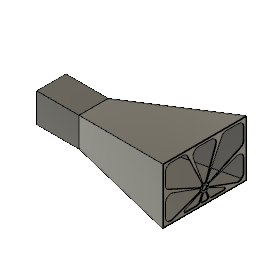
ion thruster-4 v1 (Autodesk Fusion 360 design; units mm, degrees)
Autodesk Fusion 360 part; units mm, degrees
sketch "Skizze7" plane through (0, 0, 0) normal (1, 0, 0) x (0, 1, 0)
  line L0 (-53, 53) -> (53, 53)
  line L1 (53, 53) -> (53, -53)
  line L2 (53, -53) -> (-53, -53)
  line L3 (-53, -53) -> (-53, 53)
  line L4 (-53, 53) -> (53, -53) construction
  line L5 (53, 53) -> (-53, -53) construction
  dimension "d31" = 106
  dimension "d32" = 106
  constraint horizontal L0
  constraint perpendicular L0 L1
  constraint parallel L0 L2
  constraint parallel L1 L3
  constraint coincident L4 origin
  constraint coincident L5 origin
  measures "d31" distance of L1.end L2.end
  measures "d32" distance of L0.end L1.end
extrude "Extrusion4" add sketch "Skizze7" against normal blind 153 makes body 1
sketch "Skizze8" plane through (0, 0, 0) normal (1, 0, 0) x (0, 1, 0)
  line L0 (50, -50) -> (-50, -50)
  line L1 (-50, -50) -> (-50, 50)
  line L2 (-50, 50) -> (50, 50)
  line L3 (50, 50) -> (50, -50)
  line L4 (50, -50) -> (-50, 50) construction
  line L5 (-50, -50) -> (50, 50) construction
  dimension "d35" = 100
  dimension "d36" = 100
  constraint horizontal L0
  constraint perpendicular L0 L1
  constraint parallel L0 L2
  constraint parallel L1 L3
  constraint coincident L4 origin
  constraint coincident L5 origin
  measures "d35" distance of L1.end L2.end
  measures "d36" distance of L0.end L1.end
extrude "Extrusion5" cut sketch "Skizze8" against normal blind 150 bodies 1
sketch "Skizze9" plane through (-153, 0, 0) normal (-1, 0, 0) x (0, -1, 0)
  line L0 (-53, -53) -> (53, -53)
  line L1 (53, -53) -> (53, 53)
  line L2 (53, 53) -> (-53, 53)
  line L3 (-53, 53) -> (-53, -53)
  line L4 (53, 53) -> (-53, 53)
  line L5 (-53, 53) -> (-53, -53)
  line L6 (-53, -53) -> (53, -53)
  line L7 (53, -53) -> (53, 53)
  circle A0 centre (0, 0) radius 9
  line L8 (-6.1659, -16.9405) -> (-14.5398, -39.9479)
  line L9 (-16.2488, -5.9141) -> (-39.9479, -14.5398)
  line L10 (-16.9405, 6.1659) -> (-39.9479, 14.5398)
  line L11 (-5.9141, 16.2488) -> (-15.0283, 41.2899)
  line L12 (5.9141, 16.2488) -> (15.0283, 41.2899)
  line L13 (16.2488, 5.9141) -> (41.2899, 15.0283)
  line L14 (16.2488, -5.9141) -> (41.2899, -15.0283)
  line L15 (6.1659, -16.9405) -> (14.5398, -39.9479)
  line L16 (-7.6189, -16.3387) -> (-20.7673, -44.5357)
  line L17 (16.3387, -7.6189) -> (44.5357, -20.7673)
  line L18 (7.6189, -16.3387) -> (20.7673, -44.5357)
  line L19 (7.3078, 15.6715) -> (21.0366, 45.1131)
  line L20 (15.6715, 7.3078) -> (45.1131, 21.0366)
  line L21 (-15.6715, 7.3078) -> (-45.1131, 21.0366)
  line L22 (-7.3078, 15.6715) -> (-21.0366, 45.1131)
  line L23 (-42, -48) -> (-26.2052, -48)
  line L24 (-48, 8.9017) -> (-48, -8.9017)
  line L25 (-48, -26.2052) -> (-48, -42)
  line L26 (-8.9017, -48) -> (8.9017, -48)
  line L27 (26.2052, -48) -> (42, -48)
  line L28 (48, -42) -> (48, -26.2052)
  line L29 (48, -10.3298) -> (48, 10.3298)
  line L30 (48, 25.5681) -> (48, 43)
  line L31 (43, 48) -> (25.5681, 48)
  line L32 (-16.3387, -7.6189) -> (-44.5357, -20.7673)
  arc A1 (8.9335, -9.4441) -> (9.4441, -8.9335) centre (0, 0) ccw
  arc A2 (12.9703, -0.8779) -> (12.9703, 0.8779) centre (0, 0) ccw
  arc A3 (9.7922, 8.5506) -> (8.5506, 9.7922) centre (0, 0) ccw
  arc A4 (0.8779, 12.9703) -> (-0.8779, 12.9703) centre (0, 0) ccw
  arc A5 (-8.5506, 9.7922) -> (-9.7922, 8.5506) centre (0, 0) ccw
  arc A6 (-12.995, 0.3611) -> (-12.9703, -0.8779) centre (0, 0) ccw
  arc A7 (-9.4441, -8.9335) -> (-8.9335, -9.4441) centre (0, 0) ccw
  arc A8 (-0.3611, -12.995) -> (0.3611, -12.995) centre (0, 0) ccw
  arc A9 (8.9335, -9.4441) -> (7.6189, -16.3387) centre (13.0567, -13.803) ccw
  arc A10 (16.3387, -7.6189) -> (9.4441, -8.9335) centre (13.803, -13.0567) ccw
  arc A11 (48, -26.2052) -> (44.5357, -20.7673) centre (42, -26.2052) ccw
  arc A12 (20.7673, -44.5357) -> (26.2052, -48) centre (26.2052, -42) ccw
  arc A13 (42, -48) -> (48, -42) centre (42, -42) ccw
  arc A14 (6.1659, -16.9405) -> (0.3611, -12.995) centre (0.5277, -18.9927) ccw
  arc A15 (-0.3611, -12.995) -> (-6.1659, -16.9405) centre (-0.5277, -18.9927) ccw
  arc A16 (-14.5398, -39.9479) -> (-8.9017, -48) centre (-8.9017, -42) ccw
  arc A17 (8.9017, -48) -> (14.5398, -39.9479) centre (8.9017, -42) ccw
  arc A18 (-7.6189, -16.3387) -> (-8.9335, -9.4441) centre (-13.0567, -13.803) ccw
  arc A19 (-9.4441, -8.9335) -> (-16.3387, -7.6189) centre (-13.803, -13.0567) ccw
  arc A20 (-44.5357, -20.7673) -> (-48, -26.2052) centre (-42, -26.2052) ccw
  arc A21 (-48, -42) -> (-42, -48) centre (-42, -42) ccw
  arc A22 (-26.2052, -48) -> (-20.7673, -44.5357) centre (-26.2052, -42) ccw
  arc A23 (-48, -8.9017) -> (-39.9479, -14.5398) centre (-42, -8.9017) ccw
  arc A24 (-39.9479, 14.5398) -> (-48, 8.9017) centre (-42, 8.9017) ccw
  arc A25 (-12.995, 0.3611) -> (-16.9405, 6.1659) centre (-18.9927, 0.5277) ccw
  line L33 (10.3298, 48) -> (-10.3298, 48)
  line L34 (-25.5681, 48) -> (-43, 48)
  line L35 (-48, 25.5681) -> (-48, 43)
  arc A26 (-16.2488, -5.9141) -> (-12.9703, -0.8779) centre (-17.9589, -1.2156) ccw
  arc A27 (-15.6715, 7.3078) -> (-9.7922, 8.5506) centre (-13.5584, 11.8393) ccw
  arc A28 (-8.5506, 9.7922) -> (-7.3078, 15.6715) centre (-11.8393, 13.5584) ccw
  arc A29 (0.8779, 12.9703) -> (5.9141, 16.2488) centre (1.2156, 17.9589) ccw
  arc A30 (-5.9141, 16.2488) -> (-0.8779, 12.9703) centre (-1.2156, 17.9589) ccw
  arc A31 (16.2488, 5.9141) -> (12.9703, 0.8779) centre (17.9589, 1.2156) ccw
  arc A32 (7.3078, 15.6715) -> (8.5506, 9.7922) centre (11.8393, 13.5584) ccw
  arc A33 (9.7922, 8.5506) -> (15.6715, 7.3078) centre (13.5584, 11.8393) ccw
  arc A34 (12.9703, -0.8779) -> (16.2488, -5.9141) centre (17.9589, -1.2156) ccw
  arc A35 (48, 10.3298) -> (41.2899, 15.0283) centre (43, 10.3298) ccw
  arc A36 (41.2899, -15.0283) -> (48, -10.3298) centre (43, -10.3298) ccw
  arc A37 (45.1131, 21.0366) -> (48, 25.5681) centre (43, 25.5681) ccw
  arc A38 (48, 43) -> (43, 48) centre (43, 43) ccw
  arc A39 (25.5681, 48) -> (21.0366, 45.1131) centre (25.5681, 43) ccw
  arc A40 (-48, 25.5681) -> (-45.1131, 21.0366) centre (-43, 25.5681) ccw
  arc A41 (-43, 48) -> (-48, 43) centre (-43, 43) ccw
  arc A42 (-21.0366, 45.1131) -> (-25.5681, 48) centre (-25.5681, 43) ccw
  arc A43 (-10.3298, 48) -> (-15.0283, 41.2899) centre (-10.3298, 43) ccw
  arc A44 (15.0283, 41.2899) -> (10.3298, 48) centre (10.3298, 43) ccw
  dimension "d39" = 106
  dimension "d40" = 106
  dimension "d41" = 18
  dimension "d52" = 6
  dimension "d53" = 6
  dimension "d54" = 5
  dimension "d55" = 5
  constraint horizontal L4
  constraint perpendicular L4 L5
  constraint parallel L4 L6
  constraint parallel L5 L7
  constraint coincident A0.centre A1.centre
  constraint collinear L23 L26
  constraint collinear L24 L25
  constraint collinear L26 L27
  constraint collinear L28 L29
  constraint collinear L29 L30
  constraint collinear L31 L33
  constraint concentric A0 A1
  constraint concentric A1 A2
  constraint concentric A2 A3
  constraint concentric A3 A4
  constraint concentric A4 A5
  constraint concentric A5 A6
  constraint concentric A6 A7
  constraint concentric A7 A8
  constraint tangent L18 A9
  constraint tangent A1 A9
  constraint tangent A1 A10
  constraint tangent L17 A10
  constraint tangent L28 A11
  constraint tangent L17 A11
  constraint equal A10 A11
  constraint tangent L27 A12
  constraint tangent L18 A12
  constraint equal A10 A12
  constraint tangent L28 A13
  constraint tangent L27 A13
  constraint equal A10 A13
  constraint tangent L15 A14
  constraint tangent A8 A14
  constraint equal A10 A14
  constraint tangent L8 A15
  constraint tangent A8 A15
  constraint equal A10 A15
  constraint tangent L8 A16
  constraint tangent L26 A16
  constraint equal A10 A16
  constraint tangent L15 A17
  constraint tangent L26 A17
  constraint equal A10 A17
  constraint tangent L16 A18
  constraint tangent A7 A18
  constraint equal A10 A18
  constraint tangent L32 A19
  constraint tangent A7 A19
  constraint equal A10 A19
  constraint tangent L25 A20
  constraint tangent L32 A20
  constraint equal A10 A20
  constraint tangent L23 A21
  constraint tangent L25 A21
  constraint equal A10 A21
  constraint tangent L16 A22
  constraint tangent L23 A22
  constraint equal A10 A22
  constraint tangent L9 A23
  constraint tangent L24 A23
  constraint equal A10 A23
  constraint tangent L10 A24
  constraint tangent L24 A24
  constraint equal A10 A24
  constraint tangent L10 A25
  constraint tangent A6 A25
  constraint equal A10 A25
  constraint collinear L33 L34
  constraint perpendicular L34 L35
  constraint tangent L9 A26
  constraint tangent A6 A26
  constraint tangent L21 A27
  constraint tangent A5 A27
  constraint equal A26 A27
  constraint tangent L22 A28
  constraint tangent A5 A28
  constraint equal A26 A28
  constraint tangent L12 A29
  constraint tangent A4 A29
  constraint equal A26 A29
  constraint tangent L11 A30
  constraint tangent A4 A30
  constraint equal A26 A30
  constraint tangent L13 A31
  constraint tangent A2 A31
  constraint equal A26 A31
  constraint tangent L19 A32
  constraint tangent A3 A32
  constraint equal A26 A32
  constraint tangent L20 A33
  constraint tangent A3 A33
  constraint equal A26 A33
  constraint tangent L14 A34
  constraint tangent A2 A34
  constraint equal A26 A34
  constraint tangent L13 A35
  constraint tangent L29 A35
  constraint equal A26 A35
  constraint tangent L14 A36
  constraint tangent L29 A36
  constraint equal A26 A36
  constraint tangent L20 A37
  constraint tangent L30 A37
  constraint equal A26 A37
  constraint tangent L30 A38
  constraint tangent L31 A38
  constraint equal A26 A38
  constraint tangent L19 A39
  constraint tangent L31 A39
  constraint equal A26 A39
  constraint tangent L21 A40
  constraint tangent L35 A40
  constraint equal A26 A40
  constraint tangent L34 A41
  constraint tangent L35 A41
  constraint equal A26 A41
  constraint tangent L22 A42
  constraint tangent L34 A42
  constraint equal A26 A42
  constraint tangent L11 A43
  constraint tangent L33 A43
  constraint equal A26 A43
  constraint tangent L12 A44
  constraint tangent L33 A44
  measures "d39" distance of L0.start L0.end
  measures "d40" distance of L2.end L0.start
  measures "d41" diameter of A0
  measures "d52" radius of A9
  measures "d53" radius of A10
  measures "d54" radius of A26
  measures "d55" radius of A44
extrude "Extrusion6" cut sketch "Skizze9" against normal blind 3 contours A0 | L8 L15 L26 A8 A14 A15 A16 A17 | L9 L10 L24 A6 A23 A24 A25 A26 | L11 L12 A4 L33 A29 A30 A43 A44 | L13 L14 L29 A2 A31 A34 A35 A36 | L16 L23 L25 L32 A7 A18 A19 A20 A21 A22 | L17 L18 L27 L28 A1 A9 A10 A11 A12 A13 | L19 L20 L30 L31 A3 A32 A33 A37 A38 A39 | L21 L22 A5 L34 L35 A27 A28 A40 A41 A42 bodies 1
sketch "Skizze11" plane through (0, 0, 0) normal (1, 0, 0) x (0, 1, 0)
  line L0 (10, -10) -> (-10, -10)
  line L1 (-10, -10) -> (-10, 10)
  line L2 (-10, 10) -> (10, 10)
  line L3 (10, 10) -> (10, -10)
  line L4 (10, -10) -> (-10, 10) construction
  line L5 (-10, -10) -> (10, 10) construction
  dimension "d59" = 20
  dimension "d60" = 20
  constraint horizontal L0
  constraint perpendicular L0 L1
  constraint parallel L0 L2
  constraint parallel L1 L3
  constraint coincident L4 origin
  constraint coincident L5 origin
  measures "d59" distance of L1.end L2.end
  measures "d60" distance of L0.end L1.end
sketch "Skizze12" plane through (400, 0, 0) normal (1, 0, 0) x (0, 1, 0)
  line L0 (10, 10) -> (-10, 10)
  line L1 (-10, 10) -> (-10, -10)
  line L2 (-10, -10) -> (10, -10)
  line L3 (10, -10) -> (10, 10)
  line L4 (151.5, 150) -> (-151.5, 150)
  line L5 (-151.5, 150) -> (-151.5, -53)
  line L6 (-151.5, -53) -> (151.5, -53)
  line L7 (151.5, -53) -> (151.5, 150)
  dimension "d63" = 303
  dimension "d64" = 203
  dimension "d74" = 150
  dimension "d75" = 151.5
  constraint horizontal L4
  constraint perpendicular L4 L5
  constraint parallel L4 L6
  constraint parallel L5 L7
  measures "d63" distance of L5.end L6.end
  measures "d64" distance of L4.end L5.end
  measures "d74" distance of origin L4
  measures "d75" distance of L5 origin
sketch "Skizze13" plane through (0, 0, 0) normal (1, 0, 0) x (0, 1, 0)
  line L0 (53, 53) -> (-53, 53)
  line L1 (-53, 53) -> (-53, -53)
  line L2 (-53, -53) -> (53, -53)
  line L3 (53, -53) -> (53, 53)
  line L4 (53, 53) -> (-53, -53) construction
  line L5 (-53, 53) -> (53, -53) construction
  dimension "d65" = 106
  dimension "d66" = 106
  constraint horizontal L0
  constraint perpendicular L0 L1
  constraint parallel L0 L2
  constraint parallel L1 L3
  constraint coincident L4 origin
  constraint coincident L5 origin
  measures "d65" distance of L1.end L2.end
  measures "d66" distance of L0.end L1.end
loft "Erhebung1" add profiles "Skizze13", "Skizze12" section 1 section 2 separate body makes body 2
sketch "Skizze14" plane through (400, 0, 0) normal (1, 0, 0) x (0, 1, 0)
  line L0 (151.5, -53) -> (151.5, 150)
  line L1 (151.5, 150) -> (-151.5, 150)
  line L2 (-151.5, 150) -> (-151.5, -53)
  line L3 (-151.5, -53) -> (151.5, -53)
  line L4 (148.5, 147) -> (-148.5, 147)
  line L5 (-148.5, 147) -> (-148.5, -50)
  line L6 (-148.5, -50) -> (148.5, -50)
  line L7 (148.5, -50) -> (148.5, 147)
  dimension "d67" = 297
  dimension "d68" = 197
  dimension "d72" = 147
  dimension "d73" = 148.5
  constraint horizontal L4
  constraint perpendicular L4 L5
  constraint parallel L4 L6
  constraint parallel L5 L7
  measures "d67" distance of L5.end L6.end
  measures "d68" distance of L4.end L5.end
  measures "d72" distance of origin L4
  measures "d73" distance of L5 origin
sketch "Skizze15" plane through (0, 0, 0) normal (-1, 0, 0) x (0, -1, 0)
  line L0 (-53, 53) -> (-53, -53)
  line L1 (-53, -53) -> (53, -53)
  line L2 (53, -53) -> (53, 53)
  line L3 (53, 53) -> (-53, 53)
  line L4 (-50, -50) -> (50, -50)
  line L5 (50, -50) -> (50, 50)
  line L6 (50, 50) -> (-50, 50)
  line L7 (-50, 50) -> (-50, -50)
  line L8 (-50, -50) -> (50, 50) construction
  line L9 (50, -50) -> (-50, 50) construction
  dimension "d69" = 100
  dimension "d70" = 100
  constraint horizontal L4
  constraint perpendicular L4 L5
  constraint parallel L4 L6
  constraint parallel L5 L7
  constraint coincident L8 origin
  constraint coincident L9 origin
  measures "d69" distance of L5.end L6.end
  measures "d70" distance of L4.end L5.end
loft "Erhebung2" cut profiles "Skizze15", "Skizze14" section 1 contours L4 L5 L6 L7 section 2 contours L4 L5 L6 L7 bodies 2
sketch "Skizze17" plane through (400, 0, 0) normal (1, 0, 0) x (0, 1, 0)
  line L0 (148.5, 147) -> (148.5, -50)
  line L1 (148.5, -50) -> (-148.5, -50)
  line L2 (-148.5, -50) -> (-148.5, 147)
  line L3 (-148.5, 147) -> (148.5, 147)
  line L4 (151.5, -53) -> (151.5, 150)
  line L5 (151.5, 150) -> (-151.5, 150)
  line L6 (-151.5, 150) -> (-151.5, -53)
  line L7 (-151.5, -53) -> (151.5, -53)
  line L8 (-151.5, 150) -> (151.5, 150)
  line L9 (151.5, 150) -> (151.5, -53)
  line L10 (151.5, -53) -> (-151.5, -53)
  line L11 (-151.5, -53) -> (-151.5, 150)
  circle A0 centre (0, 0) radius 9
  line L12 (0, 13) -> (0, 140)
  line L13 (-5.9141, 16.2488) -> (-41.1867, 113.1596)
  line L14 (-7.3912, 15.6324) -> (-60.7793, 128.5488)
  line L15 (-16.2488, 5.9141) -> (-114.6596, 41.7327)
  line L16 (-16.2488, -5.9141) -> (-114.8277, -41.7939)
  line L17 (-15.6715, -7.3078) -> (-71.7733, -33.4685)
  line L18 (-7.3078, -15.6715) -> (-17.3589, -37.2262)
  line L19 (-5.9141, -16.2488) -> (-13.2084, -36.2899)
  line L20 (-26.4219, -43) -> (-69.6603, -43)
  line L21 (-121.6681, -43) -> (-121.5, -43)
  line L22 (-15.7102, 7.2241) -> (-129.8557, 59.7124)
  line L23 (-141.5, -23) -> (-141.5, 22.9388)
  line L24 (-141.5, 77.8833) -> (-141.5, 120)
  line L25 (-121.5, 140) -> (-78.8602, 140)
  arc A1 (-60.7793, 128.5488) -> (-78.8602, 140) centre (-78.8602, 120) ccw
  arc A2 (-121.5, 140) -> (-141.5, 120) centre (-121.5, 120) ccw
  arc A3 (-141.5, 77.8833) -> (-129.8557, 59.7124) centre (-121.5, 77.8833) ccw
  arc A4 (-141.5, -23) -> (-121.5, -43) centre (-121.5, -23) ccw
  arc A5 (-121.6681, -43) -> (-114.8277, -41.7939) centre (-121.6681, -23) ccw
  arc A6 (-114.6596, 41.7327) -> (-141.5, 22.9388) centre (-121.5, 22.9388) ccw
  arc A7 (-71.7733, -33.4685) -> (-69.6603, -43) centre (-69.6603, -38) ccw
  arc A8 (-26.4219, -43) -> (-17.3589, -37.2262) centre (-26.4219, -33) ccw
  arc A9 (-13.2084, -36.2899) -> (-8.51, -43) centre (-8.51, -38) ccw
  arc A10 (-22.3929, 140) -> (-41.1867, 113.1596) centre (-22.3929, 120) ccw
  arc A11 (-8.6027, 9.7465) -> (-9.8376, 8.4983) centre (0, 0) ccw
  arc A12 (-12.9703, 0.8779) -> (-12.9703, -0.8779) centre (0, 0) ccw
  arc A13 (-9.7922, -8.5506) -> (-8.5506, -9.7922) centre (0, 0) ccw
  arc A14 (-7.3078, -15.6715) -> (-8.5506, -9.7922) centre (-11.8393, -13.5584) ccw
  arc A15 (-9.7922, -8.5506) -> (-15.6715, -7.3078) centre (-13.5584, -11.8393) ccw
  arc A16 (-16.2488, -5.9141) -> (-12.9703, -0.8779) centre (-17.9589, -1.2156) ccw
  arc A17 (-12.9703, 0.8779) -> (-16.2488, 5.9141) centre (-17.9589, 1.2156) ccw
  arc A18 (-8.6027, 9.7465) -> (-7.3912, 15.6324) centre (-11.9114, 13.4952) ccw
  arc A19 (-15.7102, 7.2241) -> (-9.8376, 8.4983) centre (-13.6213, 11.7669) ccw
  arc A20 (-5.9141, 16.2488) -> (-0.8779, 12.9703) centre (-1.2156, 17.9589) ccw
  arc A21 (-0.8779, -12.9703) -> (-5.9141, -16.2488) centre (-1.2156, -17.9589) ccw
  arc A22 (-0.8779, -12.9703) -> (0, -13) centre (0, 0) ccw
  arc A23 (0, 13) -> (-0.8779, 12.9703) centre (0, 0) ccw
  line L26 (5.9141, 16.2488) -> (41.1867, 113.1596)
  line L27 (7.3912, 15.6324) -> (60.7793, 128.5488)
  line L28 (0, 13) -> (0, 140)
  arc A24 (78.8602, 140) -> (60.7793, 128.5488) centre (78.8602, 120) ccw
  arc A25 (41.1867, 113.1596) -> (22.3929, 140) centre (22.3929, 120) ccw
  arc A26 (141.5, 120) -> (121.5, 140) centre (121.5, 120) ccw
  line L29 (121.5, 140) -> (78.8602, 140)
  line L30 (141.5, 77.8833) -> (141.5, 120)
  arc A27 (141.5, 22.9388) -> (114.6596, 41.7327) centre (121.5, 22.9388) ccw
  line L31 (15.7102, 7.2241) -> (129.8557, 59.7124)
  line L32 (16.2488, 5.9141) -> (114.6596, 41.7327)
  arc A28 (129.8557, 59.7124) -> (141.5, 77.8833) centre (121.5, 77.8833) ccw
  line L33 (141.5, -23) -> (141.5, 22.9388)
  line L34 (15.6715, -7.3078) -> (71.7733, -33.4685)
  arc A29 (69.6603, -43) -> (71.7733, -33.4685) centre (69.6603, -38) ccw
  line L35 (26.4219, -43) -> (69.6603, -43)
  line L36 (5.9141, -16.2488) -> (13.2084, -36.2899)
  line L37 (7.3078, -15.6715) -> (17.3589, -37.2262)
  arc A30 (114.8277, -41.7939) -> (121.6681, -43) centre (121.6681, -23) ccw
  line L38 (121.6681, -43) -> (121.5, -43)
  arc A31 (17.3589, -37.2262) -> (26.4219, -43) centre (26.4219, -33) ccw
  arc A32 (8.51, -43) -> (13.2084, -36.2899) centre (8.51, -38) ccw
  line L39 (16.2488, -5.9141) -> (114.8277, -41.7939)
  arc A33 (121.5, -43) -> (141.5, -23) centre (121.5, -23) ccw
  arc A34 (0.8779, 12.9703) -> (5.9141, 16.2488) centre (1.2156, 17.9589) ccw
  arc A35 (9.8376, 8.4983) -> (15.7102, 7.2241) centre (13.6213, 11.7669) ccw
  arc A36 (9.8376, 8.4983) -> (8.6027, 9.7465) centre (0, 0) ccw
  arc A37 (7.3912, 15.6324) -> (8.6027, 9.7465) centre (11.9114, 13.4952) ccw
  arc A38 (12.9703, -0.8779) -> (16.2488, -5.9141) centre (17.9589, -1.2156) ccw
  arc A39 (12.9703, -0.8779) -> (12.9703, 0.8779) centre (0, 0) ccw
  arc A40 (16.2488, 5.9141) -> (12.9703, 0.8779) centre (17.9589, 1.2156) ccw
  arc A41 (8.5506, -9.7922) -> (7.3078, -15.6715) centre (11.8393, -13.5584) ccw
  arc A42 (8.5506, -9.7922) -> (9.7922, -8.5506) centre (0, 0) ccw
  arc A43 (15.6715, -7.3078) -> (9.7922, -8.5506) centre (13.5584, -11.8393) ccw
  arc A44 (5.9141, -16.2488) -> (0.8779, -12.9703) centre (1.2156, -17.9589) ccw
  arc A45 (0, -13) -> (0.8779, -12.9703) centre (0, 0) ccw
  arc A46 (0.8779, 12.9703) -> (0, 13) centre (0, 0) ccw
  line L40 (141.5, 120) -> (141.5, 77.8833)
  line L41 (141.5, 22.9388) -> (141.5, -23)
  line L42 (-22.3929, 140) -> (22.3929, 140)
  line L43 (78.8602, 140) -> (121.5, 140)
  line L44 (121.6681, -43) -> (121.5, -43)
  line L45 (69.6603, -43) -> (26.4219, -43)
  line L46 (8.51, -43) -> (-8.51, -43)
  dimension "d93" = 18
  dimension "d104" = 20
  dimension "d105" = 20
  dimension "d106" = 20
  dimension "d107" = 20
  dimension "d108" = 20
  dimension "d109" = 5
  dimension "d110" = 10
  dimension "d111" = 5
  dimension "d112" = 20
  dimension "d113" = 5
  dimension "d114" = 5
  dimension "d115" = 5
  constraint horizontal L8
  constraint vertical L9
  constraint horizontal L10
  constraint vertical L11
  constraint coincident L4.start L7.end
  constraint coincident L5.end L6.start
  constraint coincident A0.centre A11.centre
  constraint collinear L20 L44
  constraint collinear L20 L21
  constraint collinear L23 L24
  constraint collinear L25 L42
  constraint coincident L12.end L25
  constraint coincident L12.start A12
  constraint coincident A22.end A12
  constraint tangent L25 A1
  constraint tangent L14 A1
  constraint tangent L25 A2
  constraint tangent L24 A2
  constraint tangent L22 A3
  constraint tangent L24 A3
  constraint equal A2 A3
  constraint tangent L21 A4
  constraint tangent L23 A4
  constraint tangent L16 A5
  constraint tangent L21 A5
  constraint tangent L15 A6
  constraint tangent L23 A6
  constraint tangent L17 A7
  constraint tangent L20 A7
  constraint tangent L18 A8
  constraint tangent L20 A8
  constraint tangent L19 A9
  constraint tangent A9 L44
  constraint tangent L13 A10
  constraint tangent A10 L42
  constraint concentric A0 A12
  constraint concentric A11 A12
  constraint concentric A12 A13
  constraint concentric A13 A22
  constraint tangent L18 A14
  constraint tangent A13 A14
  constraint tangent L17 A15
  constraint tangent A13 A15
  constraint tangent L16 A16
  constraint tangent A12 A16
  constraint equal A15 A16
  constraint tangent L15 A17
  constraint tangent A12 A17
  constraint equal A15 A17
  constraint tangent L14 A18
  constraint tangent A11 A18
  constraint equal A15 A18
  constraint tangent L22 A19
  constraint tangent A11 A19
  constraint equal A15 A19
  constraint tangent L13 A20
  constraint tangent A20 A22
  constraint equal A15 A20
  constraint tangent L19 A21
  constraint tangent A21 A22
  constraint concentric A22 A23
  constraint collinear L40 L41
  constraint collinear L42 L43
  constraint collinear L44 L45
  constraint collinear L45 L46
  measures "d93" diameter of A0
  measures "d104" radius of A1
  measures "d105" radius of A2
  measures "d106" radius of A4
  measures "d107" radius of A5
  measures "d108" radius of A6
  measures "d109" radius of A7
  measures "d110" radius of A8
  measures "d111" radius of A9
  measures "d112" radius of A10
  measures "d113" radius of A14
  measures "d114" radius of A15
  measures "d115" radius of A21
extrude "Extrusion8" add sketch "Skizze17" against normal blind 3 separate body contours L0 L1 L2 L3 makes body 3
equation "d73 = ( 297 / 2 ) * 1 mm"
equation "d75 = ( 303 / 2 ) * 1 mm"
